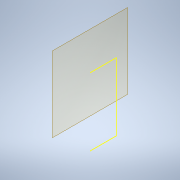
# Autodesk Inventor part: bracket
Saved by Autodesk Inventor 2020 (Build 240168000, 168)
## iProperties
Created: 2019-05-07
Part Number: bracket
Material: Generic
Document SubType Name: Modeling
Designer: erwin
Density: 1 g/cm^3
Appearance: Default
Author: erwin
Autodesk Inventor part; units mm, degrees
ref_plane "XZ Plane" through (0, 0, 0) normal (0, 1, 0) x (-1, 0, 0)
ref_plane "XY Plane" through (0, 0, 0) normal (0, 0, 1) x (1, 0, 0)
ref_plane "Work Plane1" through (-15.5, 0, 0) normal (1, 0, 0) x (0, 1, 0)
sketch "Sketch1" plane through (-15.5, 0, 0) normal (1, 0, 0) x (0, 1, 0)
  line L0 (0, 0) -> (0, -7) projected
  line L1 (0, -7) -> (-16, -7) projected
  line L2 (-18, -7) -> (-16, -7) projected
  line L3 (-18, 0) -> (-18, -7) projected
  line L4 (-18, 0) -> (-22, 0)
  line L5 (-22, 0) -> (-22, 19.5)
  line L6 (-22, 19.5) -> (-29, 19.5)
  line L7 (-29, 19.5) -> (-29, -2)
  line L8 (-29, -2) -> (-20, -2)
  line L9 (-20, -2) -> (-20, -9)
  line L10 (-20, -9) -> (2, -9)
  line L11 (-18, -7) -> (0, -7) construction
  line L12 (-9, -7) -> (-9, -16.2011) construction
  line L13 (2, -9) -> (2, -2)
  line L14 (2, -2) -> (25.8, -2)
  line L15 (25.8, -2) -> (25.8, 19.5)
  line L16 (25.8, 19.5) -> (18.8, 19.5)
  line L17 (18.8, 19.5) -> (18.8, 0)
  line L18 (18.8, 0) -> (0, 0)
  line L19 (-14, -2) -> (-14, -5) construction
  dimension "d1" = 19.5
  dimension "d2" = 2
  dimension "d3" = 2
  dimension "d4" = 2
  dimension "d5" = 7
  dimension "d6" = 7
  dimension "d7" = 2
  dimension "d8" = 8
  dimension "d9" = 40.8
  constraints: 30 end point, 11 perpendicular, 2 vertical, 1 collinear, 1 horizontal, 1 midpoint
  measures "d1" distance of L4.end L5.end
  measures "d2" distance between parallel lines of L1 L10
  measures "d3" distance between parallel lines of L3 L9
  measures "d4" distance between parallel lines of L4 L8
  measures "d5" distance of L5.end L6.end
  measures "d6" distance of L15.end L16.end
  measures "d7" distance between parallel lines of L0 L13
  measures "d8" distance between parallel lines of L5 L19
  measures "d9" distance between parallel lines of L17 L5
extrude "Extrusion1" add sketch "Sketch1" along normal blind 15
sketch "Sketch2" plane through (-0.5, 0, 0) normal (1, 0, 0) x (0, 0, -1)
  line L0 (0, -18) -> (0, -22) projected
  line L1 (0, 18.8) -> (0, 0) projected
  line L2 (-19.5, -29) -> (2, -29) projected
  line L3 (2, 25.8) -> (-19.5, 25.8) projected
  point P0 (-4.5, -25.6)
  point P1 (-14, -25.6)
  point P2 (-4.5, 22.4)
  point P3 (-14, 22.4)
  dimension "d12" = 4.5
  dimension "d13" = 9.5
  dimension "d14" = 4.5
  dimension "d15" = 9.5
  dimension "d16" = 48
  dimension "d17" = 3.4
  dimension "d18" = 3.4
  measures "d12" distance from line of L0 point (-4.5, -25.6)
  measures "d13" distance of point (-14, -25.6) point (-4.5, -25.6)
  measures "d14" distance from line of L1 point (-4.5, 22.4)
  measures "d15" distance of point (-4.5, 22.4) point (-14, 22.4)
  measures "d16" distance of point (-4.5, 22.4) point (-4.5, -25.6)
  measures "d17" distance from line of L2 point (-4.5, -25.6)
  measures "d18" distance from line of L3 point (-4.5, 22.4)
hole "Hole1" at (-0.5, -25.6, 4.5) at (-0.5, -25.6, 14) at (-0.5, 22.4, 4.5) at (-0.5, 22.4, 14) direction (-1, 0, 0) diameter 2.5 end through all
fillet "Fillet1" radius 2 8 edges at (-8, 25.8, 19.5) (-8, 25.8, -2) (-8, 2, -2) (-8, 2, -9) (-8, -20, -9) (-8, -29, -2) (-8, -29, 19.5) (-8, -20, -2)
equation "\"d2\" = d3"
equation "\"d4\" = d3"
equation "\"d7\" = d3"
equation "\"d14\" = d12"
equation "\"d15\" = d13"
equation "\"d18\" = d17"
body "Solid1"
